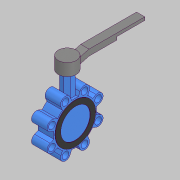
# Autodesk Inventor part: BUTTERFLY VALVE MANUAL LUG TYPE DN100
Saved by Autodesk Inventor 2017 (Build 210142000, 142)
## iProperties
Created: 2017-11-22
Part Number: BUTTERFLY VALVE MANUAL LUG TYPE DN100
Material: GG25
Document SubType Name: Modeling
Designer: Demarec
Density: 7.85 g/cm^3
Appearance: Steel - Cast(1)
Description: BELVEN BV12
Catalog Web Link: http://www.pocketbrewery.com
Author: Demarec
Autodesk Inventor part; units mm, degrees
ref_plane "YZ Plane" through (0, 0, 0) normal (1, 0, 0) x (0, 1, 0)
ref_plane "XZ Plane" through (0, 0, 0) normal (0, 1, 0) x (-1, 0, 0)
ref_plane "XY Plane" through (0, 0, 0) normal (0, 0, 1) x (1, 0, 0)
sketch "Sketch1" plane through (0, 0, 0) normal (0, 1, 0) x (-1, 0, 0)
  circle A0 centre (0, 0) radius 72.5
  circle A1 centre (0, 0) radius 77.5
  circle A2 centre (0, 0) radius 53.5
  circle A3 centre (0, 0) radius 90 construction
  line L0 (0, 0) -> (-34.4415, 83.1492) construction
  circle A4 centre (-34.4415, 83.1492) radius 12
  line L1 (0, 154) -> (-32.5, 154)
  line L2 (-32.5, 154) -> (-32.5, 198)
  line L3 (-32.5, 198) -> (0, 198)
  line L4 (0, 198) -> (0, 154)
  line L5 (0, 140.825) -> (0, 198)
  line L6 (20, 74.8749) -> (-20, 74.8749)
  line L7 (-20, 74.8749) -> (-20, 154)
  line L8 (-20, 154) -> (20, 154)
  line L9 (20, 154) -> (20, 74.8749)
  line L10 (0, 0) -> (0, 198)
  line L11 (265, 193) -> (63.4449, 193)
  line L12 (63.4449, 193) -> (63.4449, 171)
  line L13 (63.4449, 171) -> (265, 171)
  line L14 (265, 171) -> (265, 193)
  line L15 (63.4449, 193) -> (0, 176)
  line L16 (63.4449, 171) -> (0, 154)
  line L17 (0, 154) -> (0, 176)
  arc A5 (-17.8117, 90.0375) -> (-51.0713, 76.2609) centre (-34.4415, 83.1492) ccw
  line L18 (-51.0713, 76.2609) -> (-45.4768, 62.7544)
  line L19 (-20, 74.8749) -> (-20, 106.132)
  line L20 (3.012, 3.8335) -> (-33.2222, -83.6438) construction
  line L21 (265, 182) -> (164.2224, 182)
  line L22 (164.2224, 182) -> (164.2224, 171)
  line L23 (164.2224, 171) -> (265, 171)
  line L24 (265, 171) -> (265, 182)
  line L25 (-17.8117, 90.0375) -> (-12.2171, 76.531)
  line L26 (-45.4768, 62.7544) -> (-12.2171, 76.531)
  point P0 (-41.2493, -65.6106)
  point P1 (-7.6728, -77.1192)
  dimension "oDiaGasket" = 145
  dimension "oDiaOutside" = 155
  dimension "oDiaInside" = 107
  dimension "oHoledia" = 24
  dimension "oStemThick" = 40
  dimension "oAngleFirstBolt" = 22.5
  dimension "oKcircle" = 180
  dimension "oDiaTop" = 65
  dimension "oHeightTop" = 44
  dimension "oHandleLenght" = 265
  dimension "d10" = 5
  dimension "d11" = 15
  dimension "d13" = 6
  dimension "oCenterTop" = 198
  dimension "d32" = 22.5
  constraints: 54 end point, 11 parallel, 9 point on circle, 6 centre point, 5 perpendicular, 4 coincident, 4 horizontal, 4 midpoint, 3 collinear, 3 point on line, 2 tangent, 1 concentric
  measures "oDiaGasket" diameter of A0
  measures "oDiaOutside" diameter of A1
  measures "oDiaInside" diameter of A2
  measures "oHoledia" diameter of A4
  measures "oStemThick" distance between parallel lines of L9 L7
  measures "oAngleFirstBolt" angle of L0 L7
  measures "oKcircle" diameter of A3
  measures "oDiaTop" diameter of L2 L10
  measures "oHeightTop" distance of L1.end L2.end
  measures "oHandleLenght" distance from line of L3.end L14
  measures "d10" distance between parallel lines of L11 L3
  measures "d11" angle of L15 L11
  measures "d13" radial gap between concentric circles of A5 A4
  measures "oCenterTop" distance from line of L3 point (0, 0)
  measures "d32" angle of L10 L20
sketch "Sketch2" plane through (0, 0, 0) normal (0, 1, 0) x (-1, 0, 0)
  circle A0 centre (0, 0) radius 77.5
  circle A1 centre (0, 0) radius 53.5
  circle A2 centre (0, 0) radius 72.5
  circle A3 centre (0, 0) radius 53.5 projected
  circle A4 centre (0, 0) radius 72.5 projected
  circle A5 centre (0, 0) radius 77.5 projected
  constraints: 4 coincident, 3 centre point, 3 concentric
extrude "Extrusion4" add sketch "Sketch2" along normal mid plane 56 contours A0 | A2
extrude "Extrusion5" add sketch "Sketch2" along normal mid plane 60 contours A2
extrude "Extrusion8" add sketch "Sketch1" along normal mid plane 56 contours A2 | L26 A1 L6 | L6 A1 L26 | L7 A5 L25 A1 | A1 L18 A5 L7 picked at (-33.064, 68.4842) picked at (-14.4207, 75.8246)
pattern_circular "Circular Pattern2" count 8 over 360 about axis through (0, 0, 0) along (0, 1, 0) of "Extrusion8"
extrude "Extrusion6" add sketch "Sketch1" along normal mid plane 40 contours A1 L10 L5 L8 L9 | A1 L25 A5 L7 L1 L5 L10 | L7 A5 L25 A1
revolve "Revolution1" add sketch "Sketch1" angle 360 about axis through (0, 0, 0) along (0, 0, 1) contours L1 L2 L3 L4
mirror "Mirror1" about plane through (0, 0, 0) normal (1, 0, 0) of "Extrusion8"
extrude "Extrusion9" add sketch "Sketch1" along normal mid plane 30 contours L4 L15 L12 L16 | L12 L11 L14 L21 L22 L13
chamfer "Chamfer1" distance 12 angle 45 4 edges at (-20, 20, 123.9468) (20, 20, 123.9468) (-20, -20, 123.9468) (20, -20, 123.9468)
equation "\"d32\" = oAngleFirstBolt"
equation "\"d25\" = oStemThick"
body "Solid2"
